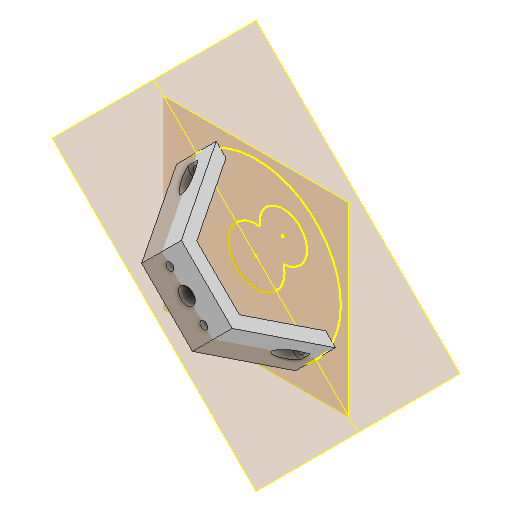
# Autodesk Inventor part: Anglerfish_Lightplate_Tislinkbridge
Saved by Autodesk Inventor 2022 (Build 260153000, 153)
## iProperties
Created: 2022-08-14
Part Number: Anglerfish_Lightplate_Tislinkbridge
Material: Generic
Document SubType Name: Modeling
Designer: diederichbenedict
Density: 1 g/cm^3
Appearance: Default
Author: diederichbenedict
Autodesk Inventor part; units mm, degrees
ref_plane "YZ Plane" through (0, 0, 0) normal (1, 0, 0) x (0, 1, 0)
ref_plane "XZ Plane" through (0, 0, 0) normal (0, 1, 0) x (-1, 0, 0)
ref_plane "XY Plane" through (0, 0, 0) normal (0, 0, 1) x (1, 0, 0)
ref_plane "Work Plane1" through (0, 0, 0) normal (0, 0, 1) x (1, 0, 0)
sketch "Sketch1" plane through (0, 0, 0) normal (0, 0, 1) x (1, 0, 0)
  circle A0 centre (18.3844, -18.3844) radius 1.4 projected
  circle A1 centre (-18.3822, 18.3822) radius 1.4 projected
  arc A2 (9.6814, 2.5019) -> (1.0662, 9.9409) centre (9.4999, 11) ccw projected
  arc A3 (1.0662, 9.9409) -> (9.6814, 2.5019) centre (0, -0.0021) ccw projected
  circle A4 centre (0, 0) radius 30 projected
ref_plane "Work Plane3" through (18.3844, -18.3844, 0) normal (0.7071, 0.7071, 0) x (-0.7071, 0.7071, 0)
ref_plane "Work Plane2" through (0, 0, 0) normal (0, 0, 1) x (1, 0, 0)
sketch "Sketch2" plane through (18.3844, -18.3844, 0) normal (0.7071, 0.7071, 0) x (-0.7071, 0.7071, 0)
  line L0 (55.9994, 0) -> (-4.0006, 0) projected
  line L1 (-4.0006, 0) -> (13.2067, 24.5746)
  line L2 (-4.0006, 0) -> (25.9994, 0) construction
  line L3 (22.8954, 10) -> (30.4529, 10) projected
  line L4 (-36.9123, 0) -> (106.4847, 0) projected
  line L5 (55.9994, 0) -> (38.7921, 24.5746)
  line L6 (55.9994, 0) -> (85.9994, 0) construction
  line L7 (38.7921, 24.5746) -> (13.2067, 24.5746)
  line L8 (0.8825, 0) -> (15.289, 20.5746)
  line L9 (15.289, 20.5746) -> (36.7098, 20.5746)
  line L10 (36.7098, 20.5746) -> (51.1163, 0)
  line L11 (55.9994, 0) -> (51.1163, 0)
  line L12 (0.8825, 0) -> (-4.0006, 0)
  point P0 (25.9994, 0)
  point P1 (0.8825, 0)
  point P2 (51.1163, 0)
  dimension "d1" = 30
  dimension "d2" = 55
  dimension "d3" = 125
  dimension "d5" = 4
  dimension "d6" = 4
  dimension "d7" = 4
  constraints: 20 end point, 4 horizontal, 3 parallel, 2 equal length, 2 point on line, 1 collinear
  measures "d1" distance of L0.end L1.end
  measures "d2" angle of L2 L1
  measures "d3" angle of L6 L5
  measures "d5" distance between parallel lines of L8 L1
  measures "d6" distance between parallel lines of L5 L10
  measures "d7" distance between parallel lines of L7 L9
extrude "Extrusion1" add sketch "Sketch2" along normal mid plane 20 contours L0 L10 L9 L8 L1 L7 L5
sketch "Sketch3" plane through (16.1169, -1.9747, 24.5746) normal (0, 0, 1) x (0.7071, 0.7071, 0)
  circle A0 centre (-10, 38.7891) radius 1.4 projected
  circle A1 centre (-10, -13.2067) radius 1.4 projected
  point P0 (-10, 12.7927)
hole "Hole1" at (-18.3822, 18.3822, 24.5746) at (18.3844, -18.3844, 24.5746) direction (0, 0, -1) diameter 2.8 end through all counterbore diameter 6.5 counterbore depth 22
sketch "Sketch4" plane through (16.1169, -1.9747, 24.5746) normal (0, 0, 1) x (0.7071, 0.7071, 0)
  circle A0 centre (-10.0015, 21.2913) radius 1.9 projected
  line L0 (0, 0) -> (-20, 0) projected
  line L1 (0, 25.5854) -> (0, 0) projected
  line L2 (-20, 25.5854) -> (0, 25.5854) projected
  line L3 (-20, 0) -> (-20, 25.5854) projected
  circle A1 centre (-10.0015, 4.2912) radius 1.9 projected
  circle A2 centre (-10.0015, 12.7912) radius 3 projected
  circle A3 centre (-10.0015, 21.2913) radius 1.4
  circle A4 centre (-10.0015, 4.2912) radius 1.9
  circle A5 centre (-10.0015, 4.2912) radius 1.4
  point P0 (-10, 12.7927)
  dimension "d17" = 2.8
  dimension "d18" = 2.8
  constraints: 3 centre point, 3 coincident, 1 concentric
  measures "d17" diameter of A3
  measures "d18" diameter of A5
extrude "Extrusion2" cut sketch "Sketch4" against normal blind 20 contours A2 | A3 | A5
body "Solid1"
